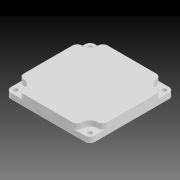
# Autodesk Inventor part: KB33-046-009 - Колпак лидара
Saved by Autodesk Inventor 2020 (Build 240168000, 168)
## iProperties
Created: 2021-08-10
Part Number: KB33-046-009 - Колпак лидара
Material: Типовые
Document SubType Name: Modeling
Designer: Петров Иван
Mass: 60.7498 g
Surface Area: 159.254 cm^2
Volume: 60.7498 cm^3
Density: 1 g/cm^3
Appearance: По умолчанию
Author: Петров Иван
Autodesk Inventor part; units mm, degrees
ref_plane "YZ Plane" through (0, 0, 0) normal (1, 0, 0) x (0, 1, 0)
ref_plane "XZ Plane" through (0, 0, 0) normal (0, 1, 0) x (-1, 0, 0)
ref_plane "XY Plane" through (0, 0, 0) normal (0, 0, 1) x (1, 0, 0)
sketch "Эскиз1" plane through (0, 0, 0) normal (0, 1, 0) x (-1, 0, 0)
  circle A0 centre (35.3553, 35.3553) radius 2
  circle A1 centre (-35.3553, 35.3553) radius 2
  circle A2 centre (-35.3553, -35.3553) radius 2
  circle A3 centre (35.3553, -35.3553) radius 2
  line L0 (-40, 40) -> (40, 40)
  line L1 (40, 40) -> (40, -40)
  line L2 (40, -40) -> (-40, -40)
  line L3 (-40, -40) -> (-40, 40)
  line L4 (-40, 40) -> (40, -40) construction
  line L5 (40, 40) -> (-40, -40) construction
  line L6 (35.3553, 35.3553) -> (0, 0) construction
  line L7 (0, 0) -> (0, 4.1405) construction
  dimension "d0" = 4
  dimension "d1" = 50
  dimension "d4" = 360
  dimension "d6" = 80
  dimension "d7" = 80
  dimension "d17" = 45
  constraints: 16 end point, 4 centre point, 2 midpoint, 2 parallel, 1 horizontal, 1 perpendicular, 1 vertical, 9 other
  measures "d0" diameter of A0
  measures "d1" distance of L6.end L6.start
  measures "d6" distance of L1.end L2.end
  measures "d7" distance of L0.end L1.end
  measures "d17" angle of L7 L6
extrude "Выдавливание1" add sketch "Эскиз1" along normal blind 10
sketch "Эскиз2" plane through (0, 10, 0) normal (0, 1, 0) x (1, 0, 0)
  circle A0 centre (-35.3553, -35.3553) radius 2 projected
  circle A1 centre (-35.3553, -35.3553) radius 7.5
  point P0 (0, 0)
  dimension "d10" = 15
  constraints: 1 centre point, 1 coincident
  measures "d10" diameter of A1
extrude "Выдавливание2" cut sketch "Эскиз2" against normal blind 5
pattern_circular "Круговой массив1" count 4 over 360 about axis through (0, -10, 0) along (0, 1, 0) of "Выдавливание2"
fillet "Сопряжение1" radius 4.75 12 edges at (29.4666, 7.5, 40) (40, 7.5, 29.4666) (40, 7.5, -29.4666) (29.4666, 7.5, -40) (-29.4666, 7.5, -40) (-40, 7.5, -29.4666) (-40, 7.5, 29.4666) (-29.4666, 7.5, 40) (-40, 2.5, 40) (40, 2.5, 40) (40, 2.5, -40) (-40, 2.5, -40)
